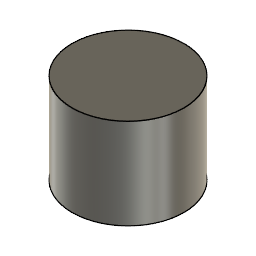
coneplayerpiece2 (Autodesk Fusion 360 archive; units mm, degrees)
design "playerbase2"
Autodesk Fusion 360 part; units mm, degrees
sketch "Sketch1" plane through (0, 0, 0) normal (0, 0, 1) x (1, 0, 0)
  circle A0 centre (0, 0) radius 2.3495
  dimension "d1" = 4.699
  constraint coincident A0.centre origin
  measures "d1" diameter of A0
extrude "Extrude1" add sketch "Sketch1" along normal blind 3.81

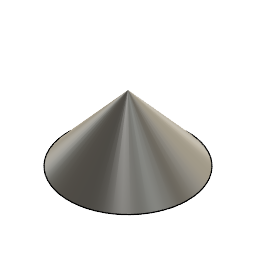
design "cone2"
Autodesk Fusion 360 part; units mm, degrees
sketch "Sketch1" plane through (0, 0, 0) normal (0, 0, 1) x (1, 0, 0)
  line L0 (0, 0) -> (22.86, 0)
  line L1 (22.86, 0) -> (22.86, 25.4)
  line L2 (0, 0) -> (22.86, 25.4)
  dimension "d1" = 22.86
  dimension "d2" = 25.4
  constraint coincident L0.start L2.start
  constraint horizontal L0
  constraint perpendicular L0 L1
  measures "d1" distance of L0.start L0.end
  measures "d2" distance of L0.end L1.end
revolve "Revolve1" add sketch "Sketch1" angle 360 about axis through (22.86, 0, 0) along (0, 1, 0)
move_body "MoveFace1" bodies 1 to x (1, 0, 0) y (0, 0, 1) z (0, -1, 0) at (0, 0, 0)
